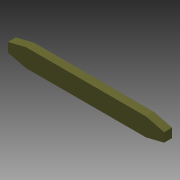
# Autodesk Inventor part: Head Bar Solid
Saved by Autodesk Inventor 2015 (Build 190159000, 159)
## iProperties
Created: 2009-06-18
Part Number: Head Bar Solid
Document SubType Name: Modeling
Designer: osbornej
Density: 4.51 g/cm^3
Material: Titanium
Mass: 0.311604 g
Surface Area: 2.3042 cm^2
Volume: 0.0690918 cm^3
Description: Head Fixed Post
Appearance: Titanium
Title: Head Fixed Post
Author: osbornej
Autodesk Inventor part; units mm, degrees
ref_plane "YZ Plane" through (0, 0, 0) normal (1, 0, 0) x (0, 1, 0)
ref_plane "XZ Plane" through (0, 0, 0) normal (0, 1, 0) x (-1, 0, 0)
ref_plane "XY Plane" through (0, 0, 0) normal (0, 0, 1) x (1, 0, 0)
sketch "Sketch1" plane through (0, 0, 0) normal (0, 0, 1) x (1, 0, 0)
  line L0 (-10.541, 1.5875) -> (10.541, 1.5875)
  line L1 (13.716, 0.7938) -> (13.716, -0.7937)
  line L2 (10.541, -1.5875) -> (-10.541, -1.5875)
  line L3 (-13.716, -0.7937) -> (-13.716, 0.7938)
  line L4 (-19.2024, 0) -> (19.2024, 0) projected
  line L5 (0, -2.2225) -> (0, 2.2225) projected
  line L6 (-10.541, 1.5875) -> (-13.716, 0.7938)
  line L7 (-10.541, -1.5875) -> (-13.716, -0.7937)
  line L8 (13.716, -0.7937) -> (10.541, -1.5875)
  line L9 (13.716, 0.7938) -> (10.541, 1.5875)
  line L10 (-0.635, 0) -> (-0.635, 0)
  line L11 (-8.255, 0) -> (-8.255, 0)
  line L12 (8.255, 0) -> (8.255, 0)
  line L13 (0.635, 0) -> (0.635, 0)
  dimension "d0" = 27.432
  dimension "d1" = 3.175
  dimension "d2" = 13.716
  dimension "d3" = 1.5875
  dimension "d5" = 3.175
  dimension "d6" = 1.5875
  dimension "d7" = 0.7937
  dimension "d8" = 1.5875
  dimension "d9" = 0.7937
  dimension "d10" = 3.175
  dimension "d11" = 3.175
  constraints: 24 end point, 5 parallel, 1 horizontal, 1 perpendicular
  measures "d0" distance between parallel lines of L1 L3
  measures "d1" distance between parallel lines of L2 L0
  measures "d2" distance between parallel lines of L1 L5
  measures "d3" distance between parallel lines of L4 L0
  measures "d5" distance from line of L1 L0.end
  measures "d6" distance of L1.end L1.start
  measures "d7" distance from line of L4 L1.end
  measures "d8" distance of L3.end L3.start
  measures "d9" distance from line of L4 L3.start
  measures "d10" horizontal distance of L2.end L3.start
  measures "d11" distance from line of L2.start L1
extrude "Extrusion2" add sketch "Sketch1" along normal blind 1.397
equation "\"d9\" = 0.5 * d8"
body "Solid2"
